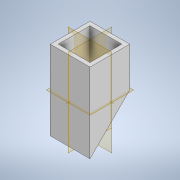
# Autodesk Inventor part: Chimney
Saved by Autodesk Inventor 2022.4 (Build 264492010, 492A)
## iProperties
Created: 2025-02-23
Part Number: Chimney
Material: Generic
Document SubType Name: Modeling
Designer: jan-m
Density: 1 g/cm^3
Appearance: Default
Author: jan-m
Autodesk Inventor part; units mm, degrees
sketch "Sketch1" plane through (0, 0, 0) normal (1, 0, 0) x (0, 1, 0)
  line L0 (20, 10) -> (-20, 10)
  line L1 (-20, 10) -> (-20, -10)
  line L2 (-20, -10) -> (20, -10)
  line L3 (20, -10) -> (20, 10)
  line L4 (-28, 0) -> (28, 0) projected
  line L5 (0, 14) -> (0, -14) projected
  line L6 (0, -10) -> (-20, 10)
  point P0 (0, 0)
  point P1 (20, 0)
  point P2 (0, 10)
  dimension "d0" = 20
  dimension "d1" = 40
  constraints: 10 end point, 3 midpoint, 3 point on line, 2 parallel, 1 horizontal, 1 perpendicular
  measures "d0" distance of L2.end L0.start
  measures "d1" distance of L0.start L0.end
extrude "Extrusion1" add sketch "Sketch1" along normal mid plane 20 contours L3 L4 L5 L0 | L5 L4 L6 L0 | L3 L2 L5 L4 | L5 L6 L4
sketch "Sketch2" plane through (-10, 20, 10) normal (0, 1, 0) x (1, 0, 0)
  line L0 (20, 20) -> (0, 20) projected
  line L1 (20, 20) -> (20, 0) projected
  line L2 (0, 0) -> (0, 20) projected
  line L3 (0, 0) -> (20, 0) projected
  line L4 (2, 18) -> (18, 18)
  line L5 (18, 18) -> (18, 2)
  line L6 (18, 2) -> (2, 2)
  line L7 (2, 2) -> (2, 18)
  point P0 (10, 10)
  dimension "d4" = 2
  constraints: 8 end point, 3 other
  measures "d4" distance between parallel lines of L0 L4
extrude "Extrusion2" cut sketch "Sketch2" against normal blind 20 contours L4 L5 L6 L7
sketch "Sketch3" plane through (10, 0, -10) normal (0, -0.7071, -0.7071) x (-1, 0, 0)
  line L0 (10, -36.7696) -> (10, 22.6274) projected
  line L1 (20, -28.2843) -> (0, -28.2843) projected
  line L2 (10, -28.2843) -> (10, 0)
  line L3 (20, 0) -> (0, 0) projected
  line L4 (10, -14.1421) -> (20, -14.1421)
  line L5 (20, -28.2843) -> (20, 0) projected
  line L6 (10, -14.1421) -> (0, -14.1421)
  circle A0 centre (5, -14.1421) radius 2.5
  line L7 (0, -28.2843) -> (0, 0) projected
  circle A1 centre (15, -14.1421) radius 2.5
  point P0 (10, -7.0711)
  point P1 (0, -14.1421)
  dimension "d8" = 5
  dimension "d9" = 5
  constraints: 6 end point, 6 midpoint, 2 centre point, 1 point on line, 1 symmetric about line, 1 other
  measures "d8" diameter of A0
  measures "d9" distance of A0.centre point (0, -14.142)
extrude "Extrusion3" cut sketch "Sketch3" against normal blind 5 contours A1 L4 | L4 A1 | A0 L6 | L6 A0
body "Solid1"
